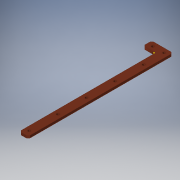
# Autodesk Inventor part: bar_+BattPow
Saved by Autodesk Inventor 2019 (Build 230136000, 136)
## iProperties
Created: 2019-05-08
Part Number: bar_+BattPow
Material: Ogólny
Document SubType Name: Modeling
Designer: Kurat
Density: 1 g/cm^3
Appearance: Miedź — satynowa
Author: Kurat
Autodesk Inventor part; units mm, degrees
ref_plane "YZ Plane" through (0, 0, 0) normal (1, 0, 0) x (0, 1, 0)
ref_plane "XZ Plane" through (0, 0, 0) normal (0, 1, 0) x (-1, 0, 0)
ref_plane "XY Plane" through (0, 0, 0) normal (0, 0, 1) x (1, 0, 0)
sketch "Szkic1" plane through (0, 0, 0) normal (0, 1, 0) x (-1, 0, 0)
  line L0 (-12.7, 166.37) -> (-12.7, -10.16)
  line L1 (-10.16, -12.7) -> (12.7, -12.7)
  line L2 (15.24, -10.16) -> (15.24, -2.54)
  line L3 (12.7, 0) -> (2.54, 0)
  line L4 (0, 2.54) -> (0, 166.37)
  line L5 (-2.54, 168.91) -> (-10.16, 168.91)
  line L6 (-6.35, 168.91) -> (-6.35, -12.7) construction
  circle A0 centre (-6.35, 161.29) radius 1.6
  circle A1 centre (-6.35, 125.73) radius 1.6
  circle A2 centre (-6.35, 90.17) radius 1.6
  circle A3 centre (-6.35, 54.61) radius 1.6
  circle A4 centre (-6.35, 19.05) radius 1.6
  line L7 (15.24, -6.35) -> (-12.7, -6.35) construction
  circle A5 centre (7.62, -6.35) radius 1.6
  circle A6 centre (-6.35, -6.35) radius 1.6
  line L8 (-2.54, 168.91) -> (0, 166.37)
  line L9 (-10.16, 168.91) -> (-12.7, 166.37)
  line L10 (-12.7, -10.16) -> (-10.16, -12.7)
  line L11 (0, 2.54) -> (2.54, 0)
  line L12 (12.7, 0) -> (15.24, -2.54)
  line L13 (12.7, -12.7) -> (15.24, -10.16)
  line L14 (-1, 165.9558) -> (-2.9542, 167.91)
  line L15 (-2.9542, 167.91) -> (-9.7458, 167.91)
  line L16 (-9.7458, 167.91) -> (-11.7, 165.9558)
  line L17 (-11.7, 165.9558) -> (-11.7, -9.7458)
  line L18 (-11.7, -9.7458) -> (-9.7458, -11.7)
  line L19 (-9.7458, -11.7) -> (12.2858, -11.7)
  line L20 (12.2858, -11.7) -> (14.24, -9.7458)
  line L21 (14.24, -9.7458) -> (14.24, -2.9542)
  line L22 (14.24, -2.9542) -> (12.2858, -1)
  line L23 (12.2858, -1) -> (2.1258, -1)
  line L24 (2.1258, -1) -> (-1, 2.1258)
  line L25 (-1, 2.1258) -> (-1, 165.9558)
  point P0 (0, 0)
  point P1 (-12.7, 168.91)
  point P2 (-12.7, -12.7)
  point P3 (15.24, -12.7)
  point P4 (15.24, 0)
  point P5 (0, 0)
  point P6 (0, 168.91)
  dimension "d0" = 12.7
  dimension "d1" = 181.61
  dimension "d2" = 27.94
  dimension "d3" = 3.2
  dimension "d4" = 7.62
  dimension "d7" = 35.56
  dimension "d12" = 3.2
  dimension "d13" = 3.2
  dimension "d14" = 7.62
  dimension "d15" = 2.54
  dimension "d16" = 2.54
  dimension "d17" = 2.54
  dimension "d18" = 2.54
  dimension "d19" = 2.54
  dimension "d20" = 2.54
  dimension "d21" = 2.54
  dimension "d22" = 2.54
  dimension "d23" = 2.54
  dimension "d24" = 2.54
  dimension "d25" = 2.54
  dimension "d26" = 2.54
  dimension "d27" = 1
  constraints: 52 end point, 18 point on line, 13 perpendicular, 7 centre point, 2 midpoint, 2 vertical, 1 coincident, 19 other
  measures "d0" distance between parallel lines of L0 L4
  measures "d1" distance between parallel lines of L1 L5
  measures "d2" distance between parallel lines of L2 L0
  measures "d3" diameter of A0
  measures "d4" distance from line of A0.centre L5
  measures "d7" distance of A0.centre A1.centre
  measures "d12" diameter of A5
  measures "d13" diameter of A6
  measures "d14" distance from line of A5.centre L2
  measures "d15" distance of L5.start point (0, 168.91)
  measures "d16" distance of L4.end point (0, 168.91)
  measures "d17" distance of L5.end point (-12.7, 168.91)
  measures "d18" distance of L0.start point (-12.7, 168.91)
  measures "d19" distance of L0.end point (-12.7, -12.7)
  measures "d20" distance of L1.start point (-12.7, -12.7)
  measures "d21" distance of L4.start point (0, 0)
  measures "d22" distance of L3.end point (0, 0)
  measures "d23" distance of L3.start point (15.24, 0)
  measures "d24" distance of L2.end point (15.24, 0)
  measures "d25" distance of L1.end point (15.24, -12.7)
  measures "d26" distance of L2.start point (15.24, -12.7)
  measures "d27" distance between parallel lines of L4 L25
extrude "Wyciągnięcie proste1" add sketch "Szkic1" along normal blind 3 contours L25 L24 L23 L22 L21 L20 L19 L18 L17 L16 L15 L14
sketch "Szkic2" plane through (0, 3, 0) normal (0, 1, 0) x (1, 0, 0)
  point P0 (0, 0)
sketch "Szkic3" plane through (0, 3, 0) normal (0, 1, 0) x (1, 0, 0)
  point P0 (0, 0)
equation "\"d16\" = d15"
equation "\"d17\" = d15"
equation "\"d18\" = d17"
equation "\"d19\" = d15"
equation "\"d20\" = d19"
equation "\"d21\" = d15"
equation "\"d22\" = d21"
equation "\"d23\" = d15"
equation "\"d24\" = d23"
equation "\"d25\" = d15"
equation "\"d26\" = d25"
